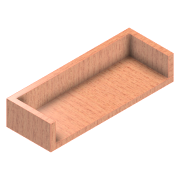
# Autodesk Inventor part: aaa
Saved by Autodesk Inventor 2021 (Build 250183000, 183)
## iProperties
Created: 2021-07-07
Part Number: aaa
Material: Generic
Document SubType Name: Modeling
Designer: Shaheen Khan
Density: 1 g/cm^3
Appearance: Red Oak - Natural Low Gloss
Author: Shaheen Khan
Autodesk Inventor part; units mm, degrees
ref_plane "YZ Plane" through (0, 0, 0) normal (1, 0, 0) x (0, 1, 0)
ref_plane "XZ Plane" through (0, 0, 0) normal (0, 1, 0) x (-1, 0, 0)
ref_plane "XY Plane" through (0, 0, 0) normal (0, 0, 1) x (1, 0, 0)
sketch "Sketch1" plane through (0, 0, 0) normal (0, 1, 0) x (-1, 0, 0)
  line L0 (-45, 125) -> (45, 125)
  line L1 (45, 125) -> (45, -125)
  line L2 (45, -125) -> (-45, -125)
  line L3 (-45, -125) -> (-45, 125)
  line L4 (-45, 125) -> (45, -125) construction
  line L5 (45, 125) -> (-45, -125) construction
  point P0 (0, 0)
  dimension "d0" = 250
  dimension "d1" = 90
  constraints: 12 end point, 2 midpoint, 2 parallel, 1 horizontal, 1 perpendicular
  measures "d0" distance of L0.end L1.end
  measures "d1" distance of L0.start L0.end
extrude "Extrusion1" add sketch "Sketch1" along normal blind 10
sketch "Sketch2" plane through (-45, 0, 125) normal (0, 0, 1) x (1, 0, 0)
  line L0 (90, 10) -> (0, 10) projected
  line L1 (0, 10) -> (90, 10)
  line L2 (90, 10) -> (90, 50)
  line L3 (90, 50) -> (0, 50)
  line L4 (0, 50) -> (0, 10)
  point P0 (45, 0)
  dimension "d4" = 40
  constraints: 8 end point, 2 parallel, 1 horizontal, 1 perpendicular
  measures "d4" distance of L1.end L2.end
extrude "Extrusion2" add sketch "Sketch2" against normal blind 10
sketch "Sketch3" plane through (45, 0, -125) normal (0, 0, -1) x (-1, 0, 0)
  line L0 (0, 0) -> (0, 50) projected
  line L1 (90, 0) -> (90, 50) projected
  line L2 (0, 9.2486) -> (90, 9.2486)
  line L3 (90, 9.2486) -> (90, 50)
  line L4 (90, 50) -> (0, 50)
  line L5 (0, 50) -> (0, 9.2486)
  point P0 (45, 0)
  point P1 (90, 9.2486)
  constraints: 8 end point, 2 parallel, 1 horizontal, 1 perpendicular, 1 point on line
extrude "Extrusion3" cut sketch "Sketch3" against normal blind 10
sketch "Sketch4" plane through (45, 0, -125) normal (0, 0, -1) x (-1, 0, 0)
  line L0 (90, 10) -> (0, 10) projected
  line L1 (90, 10) -> (90, 50) projected
  line L2 (0, 10) -> (90, 10)
  line L3 (90, 10) -> (90, 50)
  line L4 (90, 50) -> (0, 50)
  line L5 (0, 50) -> (0, 10)
  point P0 (45, 0)
  constraints: 8 end point, 2 parallel, 1 horizontal, 1 perpendicular
extrude "Extrusion4" add sketch "Sketch4" against normal blind 10
sketch "Sketch5" plane through (-45, 0, -125) normal (-1, 0, 0) x (0, 0, 1)
  line L0 (10, 50) -> (10, 10) projected
  line L1 (240, 50) -> (240, 10) projected
  line L2 (10, 10) -> (240, 10)
  line L3 (240, 10) -> (240, 50)
  line L4 (240, 50) -> (10, 50)
  line L5 (10, 50) -> (10, 10)
  point P0 (125, 0)
  constraints: 8 end point, 2 parallel, 1 horizontal, 1 perpendicular
extrude "Extrusion5" add sketch "Sketch5" against normal blind 10
body "Solid1"
